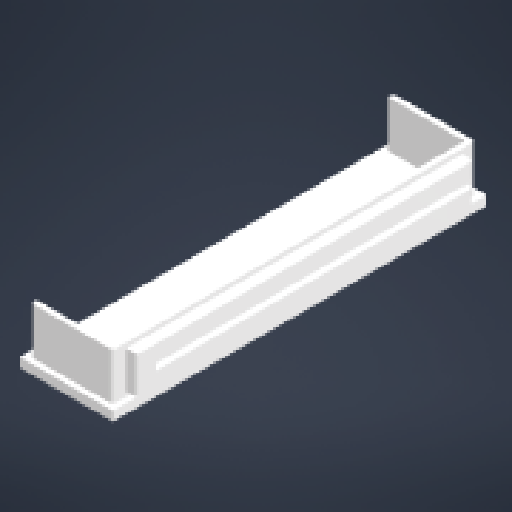
# Autodesk Inventor part: module_valve
Saved by Autodesk Inventor 2025.2 (Build 292293000, 293)
## iProperties
Created: 2025-11-09
Part Number: module_valve
Material: PC/ABS Plastic
Document SubType Name: Modeling
Designer: sam
Density: 1.1 g/cm^3
Appearance: Smooth - White
Author: sam
Autodesk Inventor part; units mm, degrees
ref_plane "YZ Plane" through (0, 0, 0) normal (1, 0, 0) x (0, 1, 0)
ref_plane "XZ Plane" through (0, 0, 0) normal (0, 1, 0) x (-1, 0, 0)
ref_plane "XY Plane" through (0, 0, 0) normal (0, 0, 1) x (1, 0, 0)
sketch "Sketch1" plane through (0, 0, 0) normal (0, 1, 0) x (-1, 0, 0)
  line L0 (-25, -100) -> (25, -100)
  line L1 (25, -100) -> (25, 100)
  line L2 (25, 100) -> (-25, 100)
  line L3 (-25, 100) -> (-25, -100)
  line L4 (-25, -100) -> (25, 100) construction
  line L5 (25, -100) -> (-25, 100) construction
  point P0 (0, 0)
  dimension "d0" = 50
  dimension "d1" = 200
  constraints: 12 end point, 2 midpoint, 2 parallel, 1 horizontal, 1 perpendicular
  measures "d0" distance of L2.end L1.end
  measures "d1" distance of L1.end L0.end
extrude "Extrusion1" add sketch "Sketch1" along normal blind 5
sketch "Sketch2" plane through (0, 5, 0) normal (0, 1, 0) x (1, 0, 0)
  line L0 (22, 97) -> (-22, 97)
  line L1 (22, -97) -> (22, 97)
  line L2 (-25, -100) -> (25, -100) projected
  line L3 (25, -100) -> (25, 100) projected
  line L4 (19, 94) -> (-22, 94)
  line L5 (19, -94) -> (19, 94)
  line L6 (25, 100) -> (-25, 100) projected
  line L7 (-22, 97) -> (-22, 94)
  line L8 (-25, 100) -> (-25, -100) projected
  line L9 (22, -97) -> (-22, -97)
  line L10 (22, -97) -> (66, -97) construction
  line L11 (19, -94) -> (-22, -94)
  line L12 (19, -94) -> (60, -94) construction
  line L13 (-22, -94) -> (-22, -97)
  point P0 (0, 0)
  dimension "d5" = 3
  dimension "d6" = 3
  dimension "d10" = 3
  dimension "d11" = 3
  dimension "d12" = 3
  dimension "d33" = 3
  dimension "d34" = 3
  dimension "d35" = 3
  constraints: 20 end point, 4 horizontal, 2 collinear, 2 vertical
  measures "d5" distance between parallel lines of L3 L1
  measures "d6" distance between parallel lines of L1 L5
  measures "d10" distance between parallel lines of L6 L0
  measures "d11" distance between parallel lines of L4 L0
  measures "d12" distance between parallel lines of L8 L7
  measures "d33" distance between parallel lines of L8 L13
  measures "d34" distance between parallel lines of L2 L9
  measures "d35" distance between parallel lines of L11 L9
extrude "Extrusion2" add sketch "Sketch2" along normal blind 25 contours L1 L9 L13 L11 L5 L4 L7 L0
fillet "Fillet1" radius 2 4 edges at (22, 17.5, 97) (22, 17.5, -97) (-22, 17.5, -97) (-22, 17.5, 97)
sketch "Sketch3" plane through (22, 5, 95) normal (1, 0, 0) x (0, 0, -1)
  line L0 (185, 22.5) -> (5, 22.5)
  line L1 (5, 22.5) -> (5, 2.5)
  line L2 (5, 2.5) -> (185, 2.5)
  line L3 (185, 2.5) -> (185, 22.5)
  line L4 (185, 22.5) -> (5, 2.5) construction
  line L5 (5, 22.5) -> (185, 2.5) construction
  line L6 (-5, -5) -> (-5, 0) projected
  line L7 (195, -5) -> (195, 0) projected
  line L8 (0, 0) -> (0, 25) projected
  point P0 (95, -5)
  point P1 (95, 12.5)
  point P2 (0, 12.5)
  dimension "d15" = 10
  dimension "d16" = 10
  dimension "d17" = 20
  dimension "d18" = 10
  constraints: 12 end point, 3 midpoint, 2 parallel, 1 horizontal, 1 perpendicular
  measures "d15" distance between parallel lines of L6 L1
  measures "d16" distance between parallel lines of L7 L3
  measures "d17" distance between parallel lines of L2 L0
  measures "d18" distance from line of point (0, 12.5) L0
extrude "Extrusion3" add sketch "Sketch3" along normal blind 6
sketch "Sketch4" plane through (22, 7.5, -90) normal (0, 0, -1) x (-1, 0, 0)
  line L0 (0, 20) -> (0, 0) projected
  line L1 (0, 20) -> (-6, 20) projected
  line L2 (-6, 0) -> (-6, 20) projected
  line L3 (0, 0) -> (-6, 0) projected
  line L4 (-6, 7.5) -> (-3, 7.5)
  line L5 (-3, 7.5) -> (-3, 12.5)
  line L6 (-3, 12.5) -> (-6, 12.5)
  line L7 (-6, 12.5) -> (-6, 7.5)
  line L8 (0, 5) -> (-3, 5)
  line L9 (-3, 5) -> (-3, 15)
  line L10 (-3, 15) -> (0, 15)
  line L11 (0, 15) -> (0, 5)
  point P0 (22, -7.5)
  point P1 (0, 15)
  point P2 (-3, 12.5)
  point P3 (-6, 12.5)
  point P4 (-3, 7.5)
  dimension "d22" = 3
  dimension "d23" = 3
  dimension "d24" = 2.5
  dimension "d25" = 2.5
  dimension "d26" = 5
  dimension "d27" = 5
  constraints: 16 end point, 4 parallel, 2 horizontal, 2 perpendicular, 2 point on line
  measures "d22" distance between parallel lines of L2 L5
  measures "d23" distance between parallel lines of L0 L9
  measures "d24" distance between parallel lines of L6 L10
  measures "d25" distance between parallel lines of L8 L4
  measures "d26" distance between parallel lines of L1 L10
  measures "d27" distance between parallel lines of L3 L8
extrude "Extrusion4" cut sketch "Sketch4" against normal blind 170 contours L0 L8 L9 L5 L10 | L6 L5 L4 L2
fillet "Fillet2" radius 2 3 edges at (28, 17.5, 90) (28, 23.75, -90) (28, 11.25, -90)
body "Solid1"
